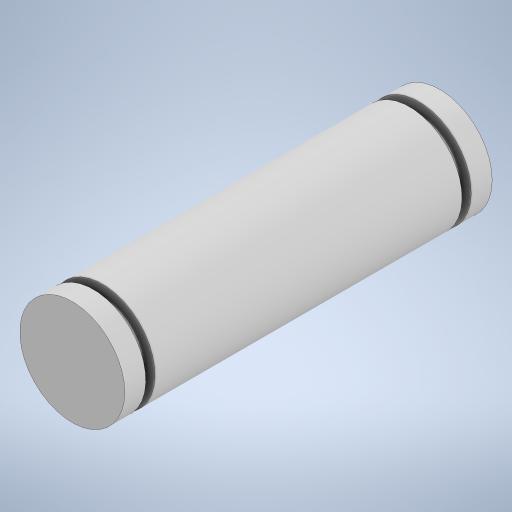
# Autodesk Inventor part: 12_Pasador
Saved by Autodesk Inventor 2024.2 (Build 282272000, 272)
## iProperties
Created: 2024-04-27
Part Number: 12_Pasador
Material: Genérico
Document SubType Name: Modeling
Designer: Cosmic Dinodog
Density: 1 g/cm^3
Appearance: Valor por defecto
Author: Cosmic Dinodog
Autodesk Inventor part; units mm, degrees
ref_plane "YZ Plane" through (0, 0, 0) normal (1, 0, 0) x (0, 1, 0)
ref_plane "XZ Plane" through (0, 0, 0) normal (0, 1, 0) x (-1, 0, 0)
sketch "Boceto1" plane through (0, 0, 0) normal (0, 0, 1) x (1, 0, 0)
  circle A0 centre (0, 0) radius 4
  dimension "d0" = 8
  constraints: 1 centre point, 1 coincident
  measures "d0" diameter of A0
extrude "Extrusión1" add sketch "Boceto1" against normal blind 28
ref_plane "Plano de trabajo1" through (0, 0, -14) normal (0, 0, 1) x (1, 0, 0)
sketch "Boceto2" plane through (0, 0, 0) normal (1, 0, 0) x (0, 1, 0)
  line L0 (0, 0) -> (0, -1.6) construction
  line L1 (0, -1.6) -> (-4, -1.6) construction
  line L2 (-4, 0) -> (-4, -28) projected
  line L3 (-4, -1.6) -> (-4, -2.3)
  line L4 (-4, -2.3) -> (-3.2, -2.3)
  line L5 (-3.2, -2.3) -> (-3.2, -1.6)
  line L6 (-4, -1.6) -> (-3.2, -1.6)
  dimension "d3" = 1.6
  dimension "d4" = 0.7
  dimension "d5" = 0.8
  constraints: 12 end point, 3 perpendicular, 3 point on line, 1 horizontal, 1 vertical
  measures "d3" distance of L0.start L0.end
  measures "d4" distance of L1.end L3.end
  measures "d5" distance of L3.end L4.end
revolve "Revolución1" cut sketch "Boceto2" angle 360 about axis through (0, 0, 0) along (0, 0, -1)
mirror "Simetría1" about plane through (0, 0, -14) normal (0, 0, 1) of "Revolución1"
